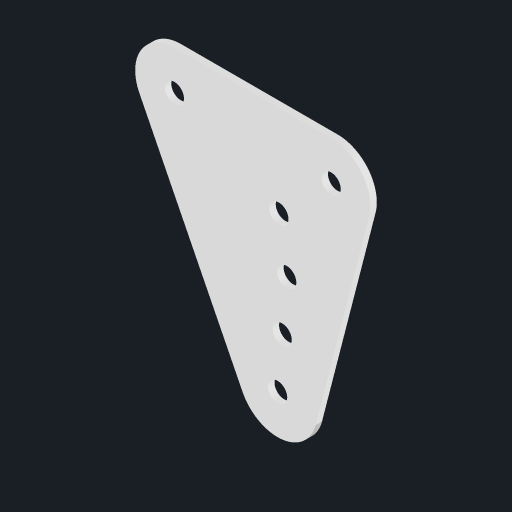
# Autodesk Inventor part: motormount
Saved by Autodesk Inventor 2024.2 (Build 282272000, 272)
## iProperties
Created: 2024-01-06
Part Number: motormount
Material: Generic
Document SubType Name: Sheet Metal
Designer: reima
Density: 1 g/cm^3
Appearance: Default
Sheet Metal Rule: Default
Author: reima
Autodesk Inventor part; units mm, degrees
ref_plane "YZ Plane" through (0, 0, 0) normal (1, 0, 0) x (0, 1, 0)
ref_plane "XZ Plane" through (0, 0, 0) normal (0, 1, 0) x (-1, 0, 0)
ref_plane "XY Plane" through (0, 0, 0) normal (0, 0, 1) x (1, 0, 0)
sketch "Sketch1" plane through (0, 0, 0) normal (0, 0, 1) x (1, 0, 0)
  circle A0 centre (-322.5487, -9.4748) radius 2.3368
  circle A1 centre (-321.4418, 3.1768) radius 2.3368
  circle A2 centre (-323.6556, -22.1265) radius 2.3368
  line L0 (-321.4418, 3.1768) -> (-321.0479, 7.6801) construction
  circle A3 centre (-367.8, 21.9203) radius 2.3114 construction
  line L1 (-378.0119, 9.2203) -> (-319.4881, 9.2203) construction
  circle A4 centre (-323.6556, -22.1265) radius 9.525
  circle A5 centre (-321.4418, 3.1768) radius 9.525
  circle A6 centre (-310.65, 28.2703) radius 2.3114 construction
  circle A7 centre (-323.35, 15.5703) radius 2.3114 construction
  circle A8 centre (-348.75, 28.2703) radius 9.525
  circle A9 centre (-310.65, 28.2703) radius 9.525
  line L2 (-332.182, -26.3721) -> (-357.2764, 24.0247)
  line L3 (-312.0866, 0.8208) -> (-311.9531, 2.3467)
  line L4 (-312.6917, -0.5863) -> (-312.0866, 0.8208)
  line L5 (-310.65, 37.7953) -> (-348.75, 37.7953)
  line L6 (-346.4386, 30.0737) -> (-346.4386, 26.4669) construction
  circle A10 centre (-348.75, 28.2703) radius 2.3114 construction
  circle A11 centre (-348.75, 28.2703) radius 2.3368
  circle A12 centre (-310.65, 28.2703) radius 2.3368
  circle A13 centre (-323.35, 15.5703) radius 2.3368
  circle A14 centre (-321.4418, 3.1768) radius 1.5848 construction
  circle A15 centre (-321.4418, 3.1768) radius 1.5848 construction
  line L7 (-314.4328, -24.5066) -> (-301.4272, 25.8902)
  point P0 (0, 0)
  point P1 (-319.4881, 34.6203)
  point P2 (-314.4552, -24.5918)
  point P3 (-301.8999, 24.5072)
  point P4 (-312.4196, 0.0464)
  dimension "d0" = 4.6736
  dimension "d1" = 4.6736
  dimension "d2" = 4.6736
  dimension "d5" = 0
  dimension "d6" = 0
  dimension "d8" = 85
  dimension "d9" = 19.05
  dimension "d10" = 19.05
  dimension "d11" = 19.05
  dimension "d12" = 19.05
  dimension "d13" = 0
  dimension "d14" = 0
  dimension "d15" = 4.6736
  dimension "d16" = 4.6736
  dimension "d17" = 4.6736
  dimension "d20" = 0
  dimension "d22" = 12.7
  dimension "d23" = 12.7
  dimension "d24" = 0
  constraints: 12 end point, 10 centre point, 10 point on circle, 10 tangent, 6 coincident, 1 other
  measures "d0" diameter of A0
  measures "d1" diameter of A1
  measures "d2" diameter of A2
  measures "d5" distance from line of L0 A0.centre
  measures "d6" distance from line of A2.centre L0
  measures "d8" angle of L1 L0
  measures "d9" diameter of A4
  measures "d10" diameter of A5
  measures "d11" diameter of A8
  measures "d12" diameter of A9
  measures "d13" distance of A8.centre A10.centre
  measures "d14" distance of A10.centre A8.centre
  measures "d15" diameter of A11
  measures "d16" diameter of A12
  measures "d17" diameter of A13
  measures "d20" distance of A14.centre L0.start
  measures "d22" distance of L0.start A0.centre
  measures "d23" distance of A0.centre A2.centre
  measures "d24" distance of A14.centre L0.start
extrude "Extrusion2" add sketch "Sketch1" along normal blind 1.5875 contours A4 | A4 L2 A8 L5 A9 L7 | A8 | A9 | A5
equation "\"BendRadius\" = Thickness"
equation "\"BendReliefWidth\" = Thickness"
equation "\"BendReliefDepth\" = 0.5 * Thickness"
equation "\"CornerReliefSize\" = 4 * Thickness"
equation "\"MinimumRemnant\" = 2 * Thickness"
equation "\"TransitionRadius\" = BendRadius"
equation "\"JacobiRadiusSize\" = BendRadius"
equation "\"GapSize\" = Thickness"
equation "\"Thickness\" = 1.5875"
body "Solid2"
